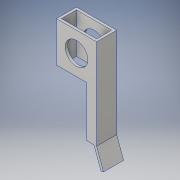
# Autodesk Inventor part: thumb block
Saved by Autodesk Inventor 2016 (Build 200138000, 138)
## iProperties
Created: 2016-02-02
Part Number: thumb block
Material: Aluminum 6061
Document SubType Name: Modeling
Designer: gus
Mass: 79.6948 g
Surface Area: 206.21 cm^2
Volume: 29.5166 cm^3
Density: 2.7 g/cm^3
Appearance: Aluminum - Flat
User Status: in process
Author: gus
Autodesk Inventor part; units mm, degrees
ref_plane "YZ Plane" through (0, 0, 0) normal (1, 0, 0) x (0, 1, 0)
ref_plane "XZ Plane" through (0, 0, 0) normal (0, 1, 0) x (-1, 0, 0)
ref_plane "XY Plane" through (0, 0, 0) normal (0, 0, 1) x (1, 0, 0)
sketch "Sketch1" plane through (0, 0, 0) normal (0, 1, 0) x (-1, 0, 0)
  line L0 (0, 0) -> (50.8, 0)
  line L1 (50.8, 0) -> (50.8, 25.4)
  line L2 (50.8, 25.4) -> (0, 25.4)
  line L3 (0, 25.4) -> (0, 0)
  line L4 (47.625, 3.175) -> (3.175, 3.175)
  line L5 (3.175, 3.175) -> (3.175, 22.225)
  line L6 (3.175, 22.225) -> (47.625, 22.225)
  line L7 (47.625, 22.225) -> (47.625, 3.175)
  dimension "d0" = 50.8
  dimension "d1" = 25.4
  dimension "d2" = 3.175
  constraints: 16 end point, 4 parallel, 2 perpendicular, 1 horizontal, 3 other
  measures "d0" distance of L2.end L1.end
  measures "d1" distance of L1.end L0.end
  measures "d2" distance between parallel lines of L0 L4
extrude "Extrusion1" add sketch "Sketch1" along normal blind 114.3
sketch "Sketch2" plane through (-50.8, 0, 25.4) normal (0, 0, 1) x (1, 0, 0)
  line L0 (0, 0) -> (38.1, 0)
  line L1 (38.1, 0) -> (38.1, 63.5)
  line L2 (38.1, 63.5) -> (0, 63.5)
  line L3 (0, 63.5) -> (0, 0)
  line L4 (0, 0) -> (50.8, 0) projected
  line L5 (0, 0) -> (0, 114.3) projected
  dimension "d5" = 38.1
  dimension "d6" = 63.5
  constraints: 8 end point, 2 collinear, 2 parallel, 1 horizontal, 1 perpendicular
  measures "d5" distance of L2.end L1.end
  measures "d6" distance of L0.end L1.end
extrude "Extrusion2" cut sketch "Sketch2" against normal blind 25.4
sketch "Sketch3" plane through (-50.8, 114.3, 25.4) normal (0, 0, 1) x (1, 0, 0)
  circle A0 centre (25.4, -25.4) radius 14.2875
  line L0 (0, 0) -> (50.8, 0) projected
  line L1 (0, -50.8) -> (0, 0) projected
  point P0 (50.8, -114.3)
  dimension "d9" = 28.575
  dimension "d10" = 25.4
  dimension "d11" = 25.4
  constraints: 1 centre point
  measures "d9" diameter of A0
  measures "d10" distance from line of L0 A0.centre
  measures "d11" distance from line of L1 A0.centre
extrude "Extrusion3" cut sketch "Sketch3" against normal blind 25.4
sketch "Sketch4" plane through (-50.8, 114.3, 25.4) normal (0, 0, 1) x (1, 0, 0)
  line L0 (50.8, -114.3) -> (59.4873, -138.1682)
  line L1 (47.4212, -114.3) -> (56.5038, -139.2541)
  line L2 (56.5038, -139.2541) -> (59.4873, -138.1682)
  line L3 (38.1, -114.3) -> (50.8, -114.3) projected
  line L4 (50.8, -114.3) -> (47.4212, -114.3)
  dimension "d14" = 25.4
  dimension "d15" = 3.175
  dimension "d16" = 110
  constraints: 8 end point, 2 perpendicular, 1 collinear, 1 horizontal
  measures "d14" distance of L0.start L0.end
  measures "d15" distance between parallel lines of L0 L1
  measures "d16" angle of L0 L3
extrude "Extrusion4" add sketch "Sketch4" against normal blind 25.4
body "Solid1"
